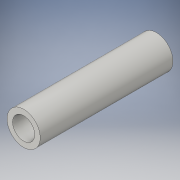
# Autodesk Inventor part: spacer
Saved by Autodesk Inventor 2016 (Build 200138000, 138)
## iProperties
Created: 2016-07-01
Part Number: spacer
Material: ABS Plastic
Document SubType Name: Modeling
Designer: rickab1
Mass: 2.44535 g
Surface Area: 17.342 cm^2
Volume: 2.30694 cm^3
Density: 1.06 g/cm^3
Appearance: Smooth - White
Author: rickab1
Autodesk Inventor part; units mm, degrees
ref_plane "YZ Plane" through (0, 0, 0) normal (1, 0, 0) x (0, 1, 0)
ref_plane "XZ Plane" through (0, 0, 0) normal (0, 1, 0) x (-1, 0, 0)
ref_plane "XY Plane" through (0, 0, 0) normal (0, 0, 1) x (1, 0, 0)
sketch "Sketch1" plane through (0, 0, 0) normal (0, 0, 1) x (1, 0, 0)
  circle A0 centre (0, 0) radius 9.525
  dimension "OD" = 19.05
  constraints: 1 centre point, 1 coincident
  measures "OD" diameter of A0
extrude "Extrusion1" add sketch "Sketch1" against normal blind 76.2
sketch "Sketch2" plane through (0, 0, 0) normal (0, 0, 1) x (1, 0, 0)
  point P0 (0, 0)
  point P1 (0, 0)
  constraints: 1 coincident
hole "Hole1" at (0, 0, 0) direction (0, 0, -1) diameter 12.7 end through all
body "Solid1"
